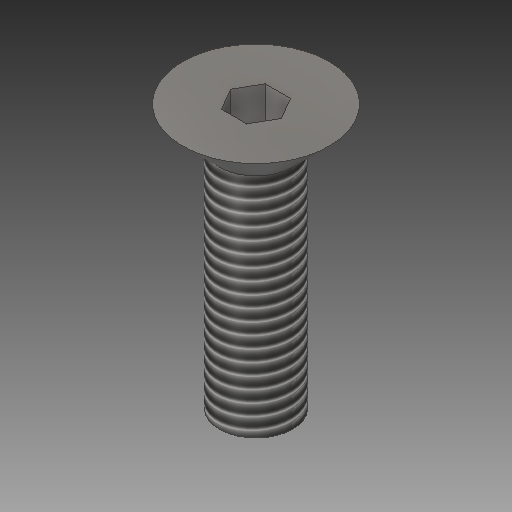
# Autodesk Inventor part: SSK-M5-18-A4
Saved by Autodesk Inventor 2019 (Build 230136000, 136)
## iProperties
Created: 2018-04-23
Part Number: SSK-M5-18-A4
Material: Stainless Steel AISI 317
Document SubType Name: Modeling
Designer: IEUser
Density: 8 g/cm^3
Appearance: Semi-Polished
Mass: 3.20762 g
Surface Area: 4.48855 cm^2
Volume: 0.400952 cm^3
Author: IEUser
Autodesk Inventor part; units mm, degrees
ref_plane "YZ Plane" through (0, 0, 0) normal (1, 0, 0) x (0, 1, 0)
ref_plane "XZ Plane" through (0, 0, 0) normal (0, 1, 0) x (-1, 0, 0)
ref_plane "XY Plane" through (0, 0, 0) normal (0, 0, 1) x (1, 0, 0)
sketch "Head Revolution Profile" plane through (0, 0, 0) normal (0, 0, 1) x (1, 0, 0)
  line L0 (0, -5) -> (5, 0)
  line L1 (5, 0) -> (0, 0)
  line L2 (0, 0) -> (0, -5)
  dimension "d0" = 0
  dimension "d1" = 45
  dimension "d2" = 5
  dimension "d3" = 0
  constraints: 6 end point, 1 horizontal, 1 perpendicular
  measures "d0" distance from line of point (0, 0) L2
  measures "d1" angle of L2 L0
  measures "d2" distance of L0.end L1.end
  measures "d3" distance from line of point (0, 0) L1
revolve "Head" add sketch "Head Revolution Profile" angle 360 about axis through (0, 0, 0) along (0, -1, 0)
sketch "Body Cross Section" plane through (0, 0, 0) normal (0, 1, 0) x (1, 0, 0)
  circle A0 centre (0, 0) radius 2.5
  point P0 (0, 0)
  dimension "d5" = 5
  constraints: 1 centre point, 1 coincident
  measures "d5" diameter of A0
extrude "Body" add sketch "Body Cross Section" against normal blind 18
thread "Thread" size "M5x0.8" class "6g" standard "ANSI Metric M Profile" full length
sketch "Key Socket Cutout Outline" plane through (0, 0, 0) normal (0, 1, 0) x (1, 0, 0)
  line L0 (0.866, 1.5) -> (1.7321, 0)
  line L1 (1.7321, 0) -> (0.866, -1.5)
  line L2 (0.866, -1.5) -> (-0.866, -1.5)
  line L3 (-0.866, -1.5) -> (-1.7321, 0)
  line L4 (-1.7321, 0) -> (-0.866, 1.5)
  line L5 (-0.866, 1.5) -> (0.866, 1.5)
  point P0 (0, 0)
  point P1 (0, 0)
  dimension "d10" = 3
  constraints: 12 end point, 1 coincident, 1 horizontal, 13 other
  measures "d10" distance between parallel lines of L2 L5
extrude "Key Socket Cutout" cut sketch "Key Socket Cutout Outline" against normal blind 2.3
body "Solid1"
